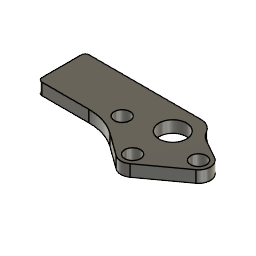
MotorMount_v4 (Autodesk Fusion 360 design; units mm, degrees)
Autodesk Fusion 360 part; units mm, degrees
sketch "Sketch1" plane through (0, 0, 0) normal (0, 0, 1) x (1, 0, 0)
  line L0 (-9.708, 0) -> (9.708, 0) construction
  line L1 (-9.708, 0) -> (0, -7.0537) construction
  line L2 (0, -7.0537) -> (9.708, 0) construction
  circle A0 centre (-9.708, 0) radius 2
  circle A1 centre (0, -7.0537) radius 2
  circle A2 centre (9.708, 0) radius 2
  line L3 (-9.708, 0) -> (0, 3.1556) construction
  line L4 (0, 3.1556) -> (9.708, 0) construction
  circle A3 centre (0, 3.1556) radius 4
  circle A4 centre (-9.708, 0) radius 3
  circle A5 centre (0, -7.0537) radius 3
  circle A6 centre (9.708, 0) radius 3
  circle A7 centre (0, 3.1556) radius 5
  line L5 (-11.1764, 2.6161) -> (-2.4473, 7.5157)
  line L6 (2.4473, 7.5157) -> (11.1764, 2.6161)
  line L7 (11.4714, -2.427) -> (1.7634, -9.4807)
  line L8 (-1.7634, -9.4807) -> (-11.4714, -2.427)
  line L9 (-11.0525, -2.7314) -> (-28.4069, -2.7314)
  line L10 (-28.4069, -2.7314) -> (-28.4069, 9.3)
  line L11 (-28.4069, 9.3) -> (4, 9.3)
  line L12 (4, 9.3) -> (4, 6.6442)
  dimension "d1" = 19.416
  dimension "d2" = 12
  dimension "d3" = 12
  dimension "d4" = 4
  dimension "d5" = 4
  dimension "d6" = 4
  dimension "d7" = 10.208
  dimension "d8" = 10.208
  dimension "d9" = 8
  dimension "d10" = 6
  dimension "d11" = 6
  dimension "d12" = 6
  dimension "d13" = 10
  constraint midpoint L0 origin
  constraint horizontal L0
  constraint coincident L0.start L1.start
  constraint coincident L1.end L2.start
  constraint coincident L0.end L2.end
  constraint coincident L3.end L4.start
  constraint concentric A0 A4
  constraint concentric A1 A5
  constraint concentric A2 A6
  constraint concentric A3 A7
  constraint coincident A4 L5.start
  constraint coincident A7 L5.end
  constraint tangent A7 L5
  constraint coincident A7 L6.start
  constraint coincident A6 L6.end
  constraint tangent A6 L6
  constraint coincident A6 L7.start
  constraint coincident A5 L7.end
  constraint tangent A5 L7
  constraint coincident A5 L8.start
  constraint coincident A4 L8.end
  constraint tangent A4 L8
  constraint tangent A5 L8
  constraint tangent A6 L7
  constraint tangent A7 L6
  constraint tangent A4 L5
  constraint coincident L8 L9.start
  constraint horizontal L9
  constraint perpendicular L9 L10
  constraint perpendicular L10 L11
  constraint coincident L6 L12.end
  constraint perpendicular L11 L12
  measures "d1" distance of L0.start L0.end
  measures "d2" distance of L0.end L1.end
  measures "d3" distance of L0.start L1.end
  measures "d4" diameter of A0
  measures "d5" diameter of A1
  measures "d6" diameter of A2
  measures "d7" distance of L0.start L3.end
  measures "d8" distance of L0.end L3.end
  measures "d9" diameter of A3
  measures "d10" diameter of A4
  measures "d11" diameter of A5
  measures "d12" diameter of A6
  measures "d13" diameter of A7
extrude "Extrude1" add sketch "Sketch1" along normal blind 3 contours A4 | A4 A5 A6 A7 L5 L6 L7 L8 | A7 | A5 | A6
move_face "OffsetFaces1" offset 0.5 1 faces at (3.995, 2.9562, 2)
extrude "Extrude2" add sketch "Sketch1" along normal blind 3 contours A4 A7 L5 L6 L8 L9 L10 L11 L12
fillet "Fillet1" radius 4.5 1 edges at (4, 6.6442, 1.5)
fillet "Fillet2" radius 4 1 edges at (4, 9.3, 1.5)
fillet "Fillet3" radius 13.5 1 edges at (-11.0525, -2.7314, 1.5)
fillet "Fillet4" radius 1 2 edges at (-28.4069, -2.7314, 1.5) (-28.4069, 9.3, 1.5)
